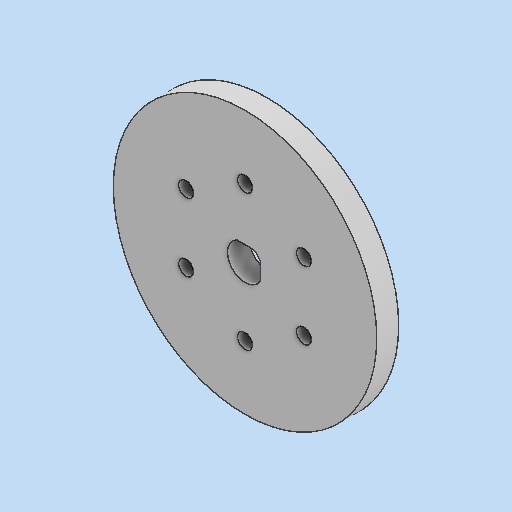
# Autodesk Inventor part: NeckInnerFlange
Saved by Autodesk Inventor 2025.2 (Build 292293000, 293)
## iProperties
Created: 2026-01-18
Part Number: NeckInnerFlange
Material: Generic
Document SubType Name: Sheet Metal
Designer: valer
Density: 1 g/cm^3
Sheet Metal Rule: Default
Appearance: Default
Author: valer
Autodesk Inventor part; units mm, degrees
ref_plane "YZ Plane" through (0, 0, 0) normal (1, 0, 0) x (0, 1, 0)
ref_plane "XZ Plane" through (0, 0, 0) normal (0, 1, 0) x (-1, 0, 0)
ref_plane "XY Plane" through (0, 0, 0) normal (0, 0, 1) x (1, 0, 0)
sketch "Base" plane through (0, 0, 0) normal (0, 0, 1) x (1, 0, 0)
  line L0 (-1.9365, 3.5) -> (1.9365, 3.5)
  arc A0 (3.5, 1.9365) -> (1.9365, 3.5) centre (0, 0) ccw
  line L1 (3.5, 1.9365) -> (3.5, -1.9365)
  arc A1 (-1.9365, 3.5) -> (3.5, -1.9365) centre (0, 0) ccw
  circle A2 centre (0, 15.5) radius 1.65 construction
  circle A3 centre (13.4234, 7.75) radius 1.65 construction
  circle A4 centre (13.4234, -7.75) radius 1.65 construction
  circle A5 centre (0, -15.5) radius 1.65 construction
  circle A6 centre (-13.4234, -7.75) radius 1.65 construction
  circle A7 centre (-13.4234, 7.75) radius 1.65 construction
  circle A8 centre (0, 0) radius 39.5
  circle A9 centre (0, 15.5) radius 1.7
  circle A10 centre (-13.4234, 7.75) radius 1.7
  circle A11 centre (-13.4234, -7.75) radius 1.7
  circle A12 centre (0, -15.5) radius 1.7
  circle A13 centre (13.4234, -7.75) radius 1.7
  circle A14 centre (13.4234, 7.75) radius 1.7
  circle A15 centre (0, 0) radius 30
  point P0 (0, 0)
  dimension "d1" = 3.4
  measures "d1" diameter of A9
extrude "Plate1" add sketch "Base" along normal blind 5 contours A15
equation "\"d0\" = Thickness"
equation "\"BendRadius\" = Thickness"
equation "\"BendReliefWidth\" = Thickness"
equation "\"BendReliefDepth\" = 0.5 * Thickness"
equation "\"TransitionRadius\" = BendRadius"
equation "\"JacobiRadiusSize\" = BendRadius"
equation "\"GapSize\" = Thickness"
equation "\"Thickness\" = 5"
body "Solid1"
